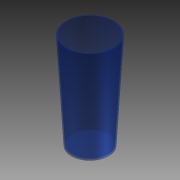
# Autodesk Inventor part: glass
Saved by Autodesk Inventor 2011 (Build 150239000, 239)
## iProperties
Created: 2013-10-30
Part Number: glass
Document SubType Name: Modeling
Designer: Devon
Density: 1 g/cm^3
Author: Devon
Autodesk Inventor part; units mm, degrees
ref_plane "YZ Plane" through (0, 0, 0) normal (1, 0, 0) x (0, 1, 0)
ref_plane "XZ Plane" through (0, 0, 0) normal (0, 1, 0) x (-1, 0, 0)
ref_plane "XY Plane" through (0, 0, 0) normal (0, 0, 1) x (1, 0, 0)
sketch "Sketch1" plane through (0, 0, 0) normal (0, 0, 1) x (1, 0, 0)
  line L0 (38.1, 114.3) -> (31.75, 0)
  line L1 (31.75, 0) -> (29.6333, -38.1)
  line L2 (29.6333, -38.1) -> (0, -38.1)
  line L3 (38.1, 114.3) -> (36.5125, 114.3)
  line L4 (36.5125, 114.3) -> (28.134, -36.5125)
  line L5 (0, -38.1) -> (0, -36.5125)
  line L6 (0, -36.5125) -> (28.134, -36.5125)
  point P0 (0, 0)
  dimension "d0" = 31.75
  dimension "d1" = 38.1
  dimension "d4" = 1.5875
  dimension "d5" = 1.5875
  constraints: 14 end point, 1 collinear, 1 parallel, 1 perpendicular
  measures "d0" distance of point (0, 0) L0.end
  measures "d1" distance of point (0, 0) L2.end
  measures "d4" distance of L0.start L3.end
  measures "d5" distance of L2.end L5.end
revolve "Revolution1" add sketch "Sketch1" angle 360 about axis through (0, -38.1, 0) along (0, 1, 0)
body "Solid1"
